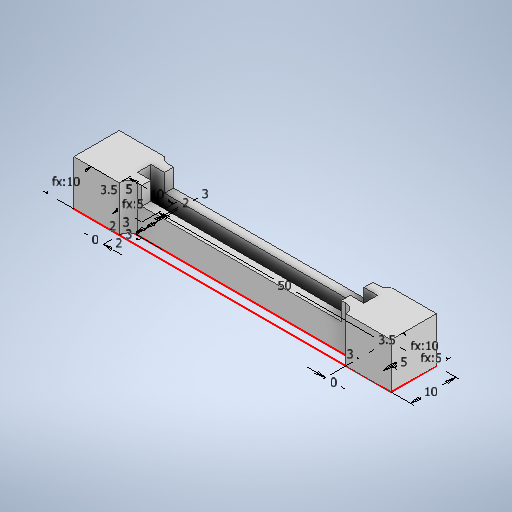
# Autodesk Inventor part: B5-camera-fu
Saved by Autodesk Inventor 2025.2 (Build 292293000, 293)
## iProperties
Created: 2025-11-05
Part Number: B5-camera-fu
Material: 일반
Document SubType Name: Modeling
Designer: RunGeun
Density: 1 g/cm^3
Appearance: 기본값
Author: RunGeun
Autodesk Inventor part; units mm, degrees
ref_plane "YZ Plane" through (0, 0, 0) normal (1, 0, 0) x (0, 1, 0)
ref_plane "XZ Plane" through (0, 0, 0) normal (0, 1, 0) x (-1, 0, 0)
ref_plane "XY Plane" through (0, 0, 0) normal (0, 0, 1) x (1, 0, 0)
sketch "스케치1" plane through (0, 0, 0) normal (0, 1, 0) x (-1, 0, 0)
  line L0 (21.7693, 2.842) -> (-28.2307, 2.842)
  line L1 (-28.2307, 2.842) -> (-28.2307, -0.158)
  line L2 (-28.2307, -0.158) -> (21.7693, -0.158)
  line L3 (21.7693, -0.158) -> (21.7693, 2.842)
  line L4 (21.7693, 4.842) -> (-28.2307, 4.842)
  line L5 (-28.2307, 4.842) -> (-28.2307, -4.158)
  line L6 (-28.2307, -4.158) -> (21.7693, -4.158)
  line L7 (21.7693, -4.158) -> (21.7693, 4.842)
  line L8 (-28.2307, 4.842) -> (-38.2307, 4.842)
  line L9 (-38.2307, 4.842) -> (-38.2307, -5.158)
  line L10 (-38.2307, -5.158) -> (-28.2307, -5.158)
  line L11 (-28.2307, -5.158) -> (-28.2307, 4.842)
  line L12 (21.7693, 4.842) -> (31.7693, 4.842)
  line L13 (31.7693, 4.842) -> (31.7693, -5.158)
  line L14 (31.7693, -5.158) -> (21.7693, -5.158)
  line L15 (21.7693, -5.158) -> (21.7693, 4.842)
  circle A0 centre (26.7693, -0.158) radius 1.75
  circle A1 centre (-33.2307, -0.158) radius 1.75
  line L16 (18.7693, 2.842) -> (18.7693, -4.158)
  line L17 (-25.2307, 2.842) -> (-25.2307, -4.158)
  line L18 (-28.2307, 0.842) -> (21.7693, 0.842)
  line L19 (21.7693, 0.842) -> (21.7693, -2.158)
  line L20 (21.7693, -2.158) -> (-28.2307, -2.158)
  line L21 (-28.2307, -2.158) -> (-28.2307, 0.842)
  point P0 (0, 0)
  point P1 (-28.2307, 2.842)
  point P2 (-25.2307, 0.842)
  point P3 (-25.2307, -2.158)
  point P4 (18.7693, -2.158)
  point P5 (18.7693, 0.842)
  dimension "d0" = 50
  dimension "d1" = 3
  dimension "d2" = 10
  dimension "d3" = 10
  dimension "d4" = 0
  dimension "d5" = 2
  dimension "d6" = 10
  dimension "d7" = 10
  dimension "d8" = 0
  dimension "d9" = 3.5
  dimension "d10" = 3.5
  dimension "d11" = 5
  dimension "d12" = 5
  dimension "d13" = 5
  dimension "d14" = 5
  dimension "d15" = 3
  dimension "d16" = 2
  dimension "d17" = 2
  dimension "d18" = 3
  dimension "d19" = 3
  constraints: 44 end point, 10 parallel, 7 perpendicular, 6 point on line, 5 horizontal, 2 centre point
  measures "d0" distance of L2.start L3.start
  measures "d1" distance of L3.start L3.end
  measures "d2" distance of L14.start L14.end
  measures "d3" distance of L10.start L11.start
  measures "d4" distance between parallel lines of L1 L5
  measures "d5" distance between parallel lines of L12 L0
  measures "d6" distance of L8.end L10.start
  measures "d7" distance of L12.end L14.start
  measures "d8" distance between parallel lines of L7 L3
  measures "d9" diameter of A1
  measures "d10" diameter of A0
  measures "d11" distance from line of A0.centre L13
  measures "d12" distance from line of A0.centre L14
  measures "d13" distance from line of A1.centre L10
  measures "d14" distance from line of A1.centre L9
  measures "d15" distance between parallel lines of L20 L18
  measures "d16" distance between parallel lines of L0 L18
  measures "d17" distance between parallel lines of L6 L20
  measures "d18" distance between parallel lines of L3 L16
  measures "d19" distance between parallel lines of L17 L1
extrude "돌출1" add sketch "스케치1" along normal blind 10 contours L7 L12 L13 L14 L15 L3 | L5 L1 L11 L10 L9 L8 | A0 | A1
extrude "돌출2" add sketch "스케치1" along normal blind 10 contours L3 L18 L16 L0 | L17 L18 L1 L0 | L7 L6 L16 L20 | L17 L6 L5 L20
extrude "돌출3" add sketch "스케치1" along normal blind 3 contours L3 L2 L16 L18 | L16 L2 L17 L18 | L7 L20 L16 L2 | L17 L2 L1 L18 | L16 L20 L17 L2 | L17 L20 L5 L2
extrude "돌출4" add sketch "스케치1" along normal blind 6 contours L16 L18 L17 L0 | L16 L6 L17 L20
fillet "모깎기1" radius 2 4 edges at (28.2307, 5, -4.158) (-21.7693, 5, -4.158) (28.2307, 5, 2.842) (-21.7693, 5, 2.842)
sketch "스케치4" plane through (28.2307, 10, -2.158) normal (-1, 0, 0) x (0, 0, 1)
  point P0 (2.158, -10)
equation "\"d3\" = d2"
equation "\"d7\" = d6"
equation "\"d12\" = d11"
equation "\"d14\" = d13"
